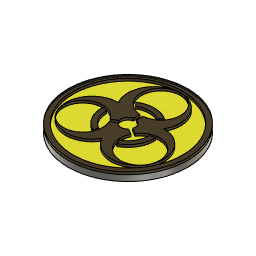
Biological Symbol v2 (Autodesk Fusion 360 design; units mm, degrees)
Autodesk Fusion 360 part; units mm, degrees
sketch "Sketch1" plane through (0, 0, 0) normal (0, 0, 1) x (1, 0, 0)
  circle A0 centre (0, 0) radius 25
  dimension "d3" = 50
  constraint coincident A0.centre origin
  measures "d3" diameter of A0
extrude "Extrude1" add sketch "Sketch1" along normal blind 2.5 makes body 1
sketch "Sketch2" plane through (0, 0, 2.5) normal (0, 0, 1) x (-1, 0, 0)
  circle A0 centre (0, 0) radius 25
  circle A1 centre (0, 0) radius 3
  circle A2 centre (0, 0) radius 9
  circle A3 centre (0, 0) radius 11
  line L0 (0, 0) -> (0, -11) construction
  circle A4 centre (0, -11) radius 11
  circle A5 centre (0, 0) radius 23
  line L1 (0, -11) -> (0, -8.2204) construction
  line L2 (0, -11) -> (0, -13.8) construction
  circle A6 centre (0, -13.8) radius 8.2
  line L3 (0.625, -5.6239) -> (-0.625, -5.6239) construction
  line L4 (-0.625, -5.6239) -> (-0.625, -2.9342)
  line L5 (0.625, -5.6239) -> (0.625, -2.9342)
  line L6 (0, -11) -> (-9.5263, 5.5) construction
  line L7 (-9.5263, 5.5) -> (9.5263, 5.5) construction
  line L8 (9.5263, 5.5) -> (0, -11) construction
  line L9 (0, 0) -> (-9.5263, 5.5) construction
  line L10 (0, 0) -> (9.5263, 5.5) construction
  line L11 (-9.5263, 5.5) -> (-11.9512, 6.9) construction
  circle A7 centre (-9.5263, 5.5) radius 11
  circle A8 centre (-11.9512, 6.9) radius 8.2
  line L12 (-5.1829, 2.2707) -> (-4.5579, 3.3532) construction
  line L13 (-5.1829, 2.2707) -> (-2.8536, 0.9258)
  line L14 (-4.5579, 3.3532) -> (-2.2286, 2.0084)
  line L15 (9.5263, 5.5) -> (11.9512, 6.9) construction
  circle A9 centre (9.5263, 5.5) radius 11
  circle A10 centre (11.9512, 6.9) radius 8.2
  line L16 (4.5579, 3.3532) -> (5.1829, 2.2707) construction
  line L17 (4.5579, 3.3532) -> (2.2286, 2.0084)
  line L18 (5.1829, 2.2707) -> (2.8536, 0.9258)
  circle A11 centre (-11.9512, 6.9) radius 7.5
  circle A12 centre (11.9512, 6.9) radius 7.5
  circle A13 centre (0, -13.8) radius 7.5
  point P0 (-9.5263, -5.5)
  dimension "d6" = 6
  dimension "d7" = 6
  dimension "d8" = 8
  dimension "d10" = 46
  dimension "d12" = 2.8
  dimension "d13" = 1.25
  dimension "d21" = 15
  constraint coincident A0.centre A1.centre
  constraint vertical L0
  constraint coincident L0.end A4.centre
  constraint concentric A1 A5
  constraint coincident A4 A0.centre
  constraint coincident L0 L1.end
  constraint parallel L0 L1
  constraint parallel L1 L2
  constraint coincident L2.end A6.centre
  constraint tangent A4 A6
  constraint coincident A6 L3.start
  constraint coincident A6 L3.end
  constraint horizontal L3
  constraint coincident A1 L4.end
  constraint perpendicular L3 L4
  constraint coincident A1 L5.end
  constraint perpendicular L3 L5
  constraint equal L6 L8
  constraint equal L6 L7
  constraint horizontal L7
  constraint equal L0 L9
  constraint parallel L9 L11
  constraint equal L2 L11
  constraint coincident L6.end L7.start
  constraint coincident A0.centre A7
  constraint coincident L11.end A8.centre
  constraint tangent A7 A8
  constraint coincident A8 L12.start
  constraint coincident A8 L12.end
  constraint perpendicular L9 L12
  constraint coincident A1 L13.end
  constraint perpendicular L12 L13
  constraint coincident A1 L14.end
  constraint perpendicular L12 L14
  constraint equal L3 L12
  constraint parallel L10 L15
  constraint equal L2 L15
  constraint coincident L7.end L8.start
  constraint coincident A0.centre A9
  constraint coincident L15.end A10.centre
  constraint tangent A9 A10
  constraint coincident A10 L16.start
  constraint coincident A10 L16.end
  constraint perpendicular L10 L16
  constraint coincident A1 L17.end
  constraint perpendicular L16 L17
  constraint coincident A1 L18.end
  constraint perpendicular L16 L18
  constraint equal L3 L16
  constraint concentric A8 A11
  constraint concentric A6 A13
  constraint equal A11 A13
  constraint equal A12 A13
  constraint coincident A7 P0
  constraint coincident A4 P0
  constraint coincident A3 P0
  measures "d6" diameter of A1
  measures "d7" distance of A1
  measures "d10" diameter of A5
  measures "d12" distance of L0.end L2.end
  measures "d13" distance of L3.start L3.end
  measures "d21" diameter of A13
extrude "Extrude2" add sketch "Sketch2" along normal blind 1 separate body contours A0 | A1 A2 A4 A10 L18 | A1 A2 A4 A9 | A1 A2 A7 A10 L17 | A1 A2 A6 L5 A9 | A2 A4 A9 | A2 A3 A4 A10 | A1 A2 A7 A9 | A2 A3 A6 A9 | A3 A4 A6 | A3 A9 A10 | A1 A2 A4 A8 L13 | A1 A2 A4 A7 | A1 A2 A6 L4 A7 | A1 A2 A8 L14 A9 | A2 A3 A7 A10 | A2 A3 A4 A8 | A2 A4 A7 | A2 A3 A6 A7 | A2 A7 A9 | A2 A3 A8 A9 | A2 A3 A12 | A3 A9 A10 | A2 A3 A13 | A3 A4 A6 | A3 A7 A8 | A3 A7 A8 | A2 A3 A11 makes body 4 at (-7.1146, 4.1076, 3.5) makes body 4 at (7.194, 4.1543, 3.5) makes body 4 at (0.0007, -8.3073, 2.5) makes body 3 at (-24.1546, 2.3847, 2.5) makes body 5 at (-9.8316, -0.7144, 3.5) makes body 6 at (4.2971, 8.8716, 2.5) makes body 2 at (5.5345, -8.1572, 2.5)
